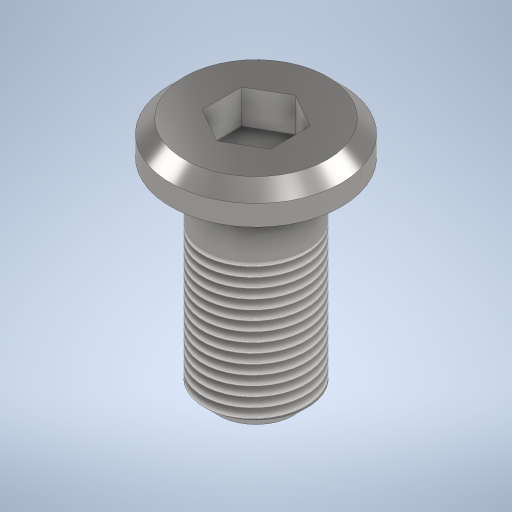
# Autodesk Inventor part: Train_003_PracticeBolt
Saved by Autodesk Inventor 2024.3 (Build 283343000, 343)
## iProperties
Created: 2026-06-11
Part Number: Train_003_PracticeBolt
Material: Stainless Steel
Document SubType Name: Modeling
Designer: scott
Density: 8 g/cm^3
Appearance: Semi-Polished
Author: scott
Autodesk Inventor part; units mm, degrees
ref_plane "YZ Plane" through (0, 0, 0) normal (1, 0, 0) x (0, 1, 0)
ref_plane "XZ Plane" through (0, 0, 0) normal (0, 1, 0) x (-1, 0, 0)
ref_plane "XY Plane" through (0, 0, 0) normal (0, 0, 1) x (1, 0, 0)
sketch "Sketch1" plane through (0, 0, 0) normal (0, 1, 0) x (-1, 0, 0)
  point P0 (0, 0)
sketch "Sketch2" plane through (0, 0, 0) normal (0, 1, 0) x (-1, 0, 0)
  circle A0 centre (0, 0) radius 1.905
  dimension "d0" = 3.81
  constraints: 1 centre point, 1 coincident
  measures "d0" diameter of A0
extrude "Extrusion1" add sketch "Sketch2" along normal blind 7.62
chamfer "Chamfer1" distance 0.508 angle 45 1 edges at (1.905, 0, 0)
sketch "Sketch3" plane through (0, 7.62, 0) normal (0, 1, 0) x (1, 0, 0)
  circle A0 centre (0, 0) radius 3.175
  dimension "d6" = 6.35
  constraints: 1 centre point, 1 coincident
  measures "d6" diameter of A0
extrude "Extrusion2" add sketch "Sketch3" along normal blind 1.27
chamfer "Chamfer2" distance 0.508 angle 45 1 edges at (-3.175, 8.89, 0)
thread "Thread1" size "M1.6x0.35" class "6g" standard "ISO Metric profile" length 5.08
sketch "Sketch4" plane through (0, 8.89, 0) normal (0, 1, 0) x (1, 0, 0)
  line L0 (0, -1.4665) -> (-1.27, -0.7332)
  line L1 (-1.27, -0.7332) -> (-1.27, 0.7332)
  line L2 (-1.27, 0.7332) -> (0, 1.4665)
  line L3 (0, 1.4665) -> (1.27, 0.7332)
  line L4 (1.27, 0.7332) -> (1.27, -0.7332)
  line L5 (1.27, -0.7332) -> (0, -1.4665)
  point P0 (0, 0)
  point P1 (0, 0)
  dimension "d14" = 2.54
  constraints: 12 end point, 1 coincident, 13 other
  measures "d14" distance between parallel lines of L1 L4
extrude "Extrusion3" cut sketch "Sketch4" against normal blind 1.27
body "Solid1"
